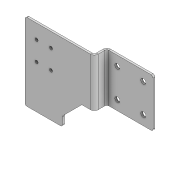
# Autodesk Inventor part: DragChain_Guide_B
Saved by Autodesk Inventor 2020 (Build 240168000, 168)
## iProperties
Created: 2021-12-05
Part Number: DragChain_Guide_B
Material: 一般
Document SubType Name: Sheet Metal
Designer: ken113
Density: 1 g/cm^3
Sheet Metal Rule: Default_mm
Appearance: 既定
Author: ken113
Autodesk Inventor part; units mm, degrees
ref_plane "YZ Plane" through (0, 0, 0) normal (1, 0, 0) x (0, 1, 0)
ref_plane "XZ Plane" through (0, 0, 0) normal (0, 1, 0) x (-1, 0, 0)
ref_plane "XY Plane" through (0, 0, 0) normal (0, 0, 1) x (1, 0, 0)
sketch "スケッチ1" plane through (0, 0, 0) normal (0, 0, 1) x (1, 0, 0)
  line L0 (25, -25) -> (-25, -25)
  line L1 (-25, -25) -> (-25, 25)
  line L2 (-25, 25) -> (25, 25)
  line L3 (25, 25) -> (25, -25)
  line L4 (25, -25) -> (-25, 25) construction
  line L5 (-25, -25) -> (25, 25) construction
  point P0 (0, 0)
  dimension "d0" = 50
  dimension "d1" = 50
  measures "d0" distance of L1.end L2.end
  measures "d1" distance of L2.end L0.start
extrude "プレート1" add sketch "スケッチ1" along normal blind 2
sketch "スケッチ2" plane through (-23, -25, 0) normal (-1, 0, 0) x (0, -1, 0)
  line L0 (-50, 0) -> (0, 0)
  line L1 (0, 0) -> (0, 15)
  line L2 (0, 15) -> (-50, 15)
  line L3 (-50, 15) -> (-50, 0)
  constraints: 6 end point, 1 horizontal, 1 perpendicular, 1 vertical
edge flange "フランジ1" height 15 angle 90 thickness 2 bend radius 2 thickness toward (-1, 0, 0) relief straight relief width 2 relief depth 1 edges at (-25, 0, 2) wall of the first edge with corners at (-23, 25, 0) (-23, -25, 0) (-23, -25, 15) (-23, 25, 15)
bend "曲げ1"
corner "コーナー1"
sketch "スケッチ3" plane through (-23, 25, 13) normal (0, 0, 1) x (1, 0, 0)
  line L0 (0, -50) -> (0, 0)
  line L1 (0, 0) -> (-72, 0)
  line L2 (-72, 0) -> (-72, -50)
  line L3 (-72, -50) -> (0, -50)
  constraints: 6 end point, 1 horizontal, 1 perpendicular, 1 vertical
edge flange "フランジ2" height 72 angle 90 thickness 2 bend radius 2 thickness toward (0, 0, 1) relief straight relief width 2 relief depth 1 edges at (-25, 0, 15) wall of the first edge with corners at (-23, -25, 13) (-23, 25, 13) (-95, 25, 13) (-95, -25, 13)
bend "曲げ2"
corner "コーナー2"
sketch "スケッチ4" plane through (0, 0, 2) normal (0, 0, 1) x (1, 0, 0)
  line L0 (-12, -15) -> (15, -15)
  line L1 (15, -15) -> (15, 15)
  line L2 (15, 15) -> (-12, 15)
  line L3 (-12, 15) -> (-12, -15)
  line L4 (-12, -15) -> (15, 15) construction
  line L5 (15, -15) -> (-12, 15) construction
  line L6 (-21, 25) -> (25, 25) projected
  line L7 (25, 25) -> (25, -25) projected
  point P0 (0, 0)
  point P1 (1.5, 0)
  dimension "d23" = 27
  dimension "d25" = 30
  dimension "d26" = 10
  dimension "d27" = 10
  constraints: 12 end point, 2 midpoint, 2 parallel, 1 horizontal, 1 perpendicular
  measures "d23" distance of L1.end L2.end
  measures "d25" distance of L0.end L1.end
  measures "d26" distance between parallel lines of L6 L2
  measures "d27" distance between parallel lines of L7 L1
hole "穴1" at (-12, 15, 2) at (-12, -15, 2) at (15, -15, 2) at (15, 15, 2) direction (0, 0, -1) diameter 5.3 depth 2 tip angle 118
fillet "フィレット1" radius 2 3 edges at (25, 25, 1) (25, -25, 1) (-95, 25, 14)
sketch "スケッチ5" plane through (-27, -25, 15) normal (0, 0, 1) x (1, 0, 0)
  line L0 (0, 0) -> (-68, 0) projected
  line L1 (0, 0) -> (0, 50) projected
  line L2 (-66, 50) -> (0, 50) projected
  arc A0 (-66, 50) -> (-68, 48) centre (-66, 48) ccw projected
  line L3 (-68, 0) -> (-68, 48) projected
  line L4 (-56, 15) -> (-41, 15)
  line L5 (-41, 15) -> (-41, 35)
  line L6 (-41, 35) -> (-56, 35)
  line L7 (-56, 35) -> (-56, 15)
  line L8 (-56, 15) -> (-41, 35) construction
  line L9 (-41, 15) -> (-56, 35) construction
  point P0 (27, 25)
  point P1 (-48.5, 25)
  dimension "d36" = 15
  dimension "d37" = 19.5
  dimension "d38" = 20
  dimension "d39" = 15
  constraints: 12 end point, 2 midpoint, 2 parallel, 1 horizontal, 1 perpendicular
  measures "d36" distance of L5.end L6.end
  measures "d37" distance from line of point (-48.5, 25) L3
  measures "d38" distance of L6.end L4.start
  measures "d39" distance between parallel lines of L2 L6
hole "穴2" at (-83, 10, 15) at (-83, -10, 15) at (-68, -10, 15) at (-68, 10, 15) direction (0, 0, -1) diameter 3.242 depth 11.8 tip angle 118 thread size "M4x0.7" class "6H" standard "ISO Metric profile"
sketch "スケッチ6" plane through (-95, -25, 15) normal (0, 0, 1) x (1, 0, 0)
  circle A0 centre (27, 15) radius 1.621 projected
  circle A1 centre (12, 35) radius 1.621 projected
  circle A2 centre (12, 15) radius 1.621 projected
  circle A3 centre (27, 35) radius 1.621 projected
  arc A4 (2, 50) -> (0, 48) centre (2, 48) ccw projected
  line L0 (0, 0) -> (0, 48) projected
  line L1 (68, 0) -> (0, 0) projected
  line L2 (68, 0) -> (68, 50) projected
  line L3 (2, 50) -> (68, 50) projected
  line L4 (0, 0) -> (39, 0)
  line L5 (39, 0) -> (39, -30)
  line L6 (39, -30) -> (0, -30)
  line L7 (0, -30) -> (0, 0)
  point P0 (95, 25)
  point P1 (39, 0)
  dimension "d47" = 39
  dimension "d48" = 80
  constraints: 8 end point, 2 parallel, 1 horizontal, 1 perpendicular
  measures "d47" distance of L5.end L6.end
  measures "d48" distance between parallel lines of L3 L6
extrude "押し出し1" add sketch "スケッチ6" against normal up to surface (2 mm away) contours L1 L5 L6 L7
chamfer "面取り1" distance 20 angle 45 1 edges at (-56, -25, 14)
fillet "フィレット2" radius 2 4 edges at (-95, -55, 14) (-56, -55, 14) (-56, -45, 14) (-36, -25, 14)
equation "\"d33\" = Thickness"
equation "\"d2\" = Thickness"
equation "\"d3\" = BendReliefWidth"
equation "\"d4\" = BendReliefDepth"
equation "\"d5\" = MinimumRemnant"
equation "\"d6\" = TransitionRadius"
equation "\"d9\" = BendRadius"
equation "\"d10\" = CornerReliefSize"
equation "\"d11\" = GapSize"
equation "\"d12\" = JacobiRadiusSize"
equation "\"d13\" = BendReliefWidth"
equation "\"d14\" = BendReliefDepth"
equation "\"d15\" = MinimumRemnant"
equation "\"d16\" = TransitionRadius"
equation "\"d19\" = BendRadius"
equation "\"d20\" = CornerReliefSize"
equation "\"d21\" = GapSize"
equation "\"d22\" = JacobiRadiusSize"
equation "\"BendRadius\" = Thickness"
equation "\"BendReliefWidth\" = Thickness"
equation "\"BendReliefDepth\" = 0.5 * Thickness"
equation "\"CornerReliefSize\" = 4 * Thickness"
equation "\"MinimumRemnant\" = 2 * Thickness"
equation "\"TransitionRadius\" = BendRadius"
equation "\"JacobiRadiusSize\" = BendRadius"
equation "\"GapSize\" = Thickness"
equation "\"Thickness\" = 2"
